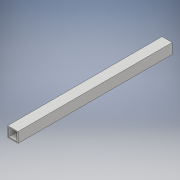
# Autodesk Inventor part: profile_alu
Saved by Autodesk Inventor 2017 (Build 210142000, 142)
## iProperties
Created: 2017-04-14
Part Number: profile_alu
Material: Generic
Document SubType Name: Modeling
Designer: franc
Density: 1 g/cm^3
Appearance: Default
Author: franc
Autodesk Inventor part; units mm, degrees
ref_plane "YZ Plane" through (0, 0, 0) normal (1, 0, 0) x (0, 1, 0)
ref_plane "XZ Plane" through (0, 0, 0) normal (0, 1, 0) x (-1, 0, 0)
ref_plane "XY Plane" through (0, 0, 0) normal (0, 0, 1) x (1, 0, 0)
sketch "Sketch1" plane through (0, 0, 0) normal (0, 1, 0) x (-1, 0, 0)
  line L0 (7.3913, 8.6413) -> (-12.6087, 8.6413)
  line L1 (-12.6087, 8.6413) -> (-12.6087, -11.3587)
  line L2 (-12.6087, -11.3587) -> (7.3913, -11.3587)
  line L3 (7.3913, -11.3587) -> (7.3913, 8.6413)
  line L4 (5.3913, 6.6413) -> (-10.6087, 6.6413)
  line L5 (-10.6087, 6.6413) -> (-10.6087, -9.3587)
  line L6 (-10.6087, -9.3587) -> (5.3913, -9.3587)
  line L7 (5.3913, -9.3587) -> (5.3913, 6.6413)
  point P0 (0, 0)
  dimension "d0" = 20
  dimension "d1" = 20
  dimension "d2" = 2
  dimension "d3" = 2
  dimension "d4" = 2
  dimension "d5" = 2
  constraints: 16 end point, 4 parallel, 2 horizontal, 2 perpendicular
  measures "d0" distance of L2.end L0.start
  measures "d1" distance of L0.start L0.end
  measures "d2" distance between parallel lines of L0 L4
  measures "d3" distance between parallel lines of L2 L6
  measures "d4" distance between parallel lines of L1 L5
  measures "d5" distance between parallel lines of L3 L7
extrude "Extrusion1" add sketch "Sketch1" along normal blind 300
body "Solid1"
